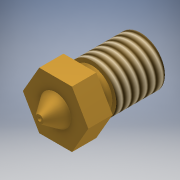
# Autodesk Inventor part: Nozzle
Saved by Autodesk Inventor 2016 (Build 200138000, 138)
## iProperties
Created: 2016-03-26
Part Number: Nozzle
Material: Brass, Soft Yellow
Document SubType Name: Modeling
Designer: Scott
Mass: 5.68329 g
Surface Area: 6.01612 cm^2
Volume: 0.67099 cm^3
Density: 8.47 g/cm^3
Appearance: Brass - Satin
Author: Scott
Autodesk Inventor part; units mm, degrees
ref_plane "YZ Plane" through (0, 0, 0) normal (1, 0, 0) x (0, 1, 0)
ref_plane "XZ Plane" through (0, 0, 0) normal (0, 1, 0) x (-1, 0, 0)
ref_plane "XY Plane" through (0, 0, 0) normal (0, 0, 1) x (1, 0, 0)
sketch "Sketch1" plane through (0, 0, 0) normal (0, 0, 1) x (1, 0, 0)
  line L0 (0, 0) -> (0.5, 0)
  line L1 (0.5, 0) -> (1.9004, 2)
  line L2 (1.9004, 2) -> (7, 2)
  line L3 (7, 2) -> (7, 5)
  line L4 (7, 5) -> (2.5, 5)
  line L5 (2.5, 5) -> (2.5, 6.5)
  line L6 (2.5, 6.5) -> (3, 6.5)
  line L7 (3, 6.5) -> (3, 12.5)
  line L8 (3, 12.5) -> (0, 12.5)
  line L9 (0, 12.5) -> (0, 0)
  dimension "d0" = 0.5
  dimension "d1" = 125
  dimension "d2" = 6
  dimension "d3" = 7.5
  dimension "d4" = 10.5
  dimension "d5" = 12.5
  dimension "d6" = 3
  dimension "d7" = 2.5
  dimension "d8" = 7
  constraints: 20 end point, 7 perpendicular, 1 horizontal, 1 parallel
  measures "d0" distance of L0.start L0.end
  measures "d1" angle of L2 L1
  measures "d2" distance between parallel lines of L6 L8
  measures "d3" distance between parallel lines of L4 L8
  measures "d4" distance between parallel lines of L2 L8
  measures "d5" distance between parallel lines of L0 L8
  measures "d6" distance of L7.end L8.end
  measures "d7" distance between parallel lines of L9 L5
  measures "d8" distance between parallel lines of L9 L3
revolve "Revolution1" add sketch "Sketch1" angle 360 about axis through (0, 12.5, 0) along (0, -1, 0)
sketch "Sketch2" plane through (0, 2, 0) normal (0, -1, 0) x (1, 0, 0)
  circle A0 centre (0, 0) radius 2.5 projected
  circle A1 centre (0, 0) radius 7 projected
  circle A2 centre (0, 0) radius 0.5 projected
  line L0 (2.0207, 3.5) -> (4.0415, 0)
  line L1 (4.0415, 0) -> (2.0207, -3.5)
  line L2 (2.0207, -3.5) -> (-2.0207, -3.5)
  line L3 (-2.0207, -3.5) -> (-4.0415, 0)
  line L4 (-4.0415, 0) -> (-2.0207, 3.5)
  line L5 (-2.0207, 3.5) -> (2.0207, 3.5)
  point P0 (0, 0)
  dimension "d10" = 7
  dimension "d11" = 3.5
  constraints: 12 end point, 1 coincident, 1 horizontal, 13 other
  measures "d10" distance between parallel lines of L2 L5
  measures "d11" distance from line of A1.centre L5
extrude "Extrusion1" cut sketch "Sketch2" against normal blind 10 contours A1
thread "Thread1" size "M6x1" class "6g" standard "ANSI Metric M Profile" full length
hole "Hole1" at (0, 12.5, 0) direction (0, -1, 0) diameter 2 depth 10.5 tip angle 118
hole "Hole2" at (0, 12.5, 0) direction (0, -1, 0) diameter 0.5 end through all
hole "Hole3" at (0, 12.5, 0) direction (0, -1, 0) diameter 1.5 depth 11.5 tip angle 118
body "Solid1"
